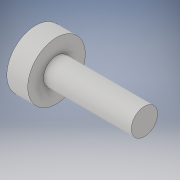
# Autodesk Inventor part: TableLEG
Saved by Autodesk Inventor 2018 (Build 220112000, 112)
## iProperties
Created: 2019-03-13
Part Number: TableLEG
Material: Generic
Document SubType Name: Modeling
Designer: 10043883
Density: 1 g/cm^3
Appearance: Default
Author: 10043883
Autodesk Inventor part; units mm, degrees
ref_plane "YZ Plane" through (0, 0, 0) normal (1, 0, 0) x (0, 1, 0)
ref_plane "XZ Plane" through (0, 0, 0) normal (0, 1, 0) x (-1, 0, 0)
ref_plane "XY Plane" through (0, 0, 0) normal (0, 0, 1) x (1, 0, 0)
sketch "Sketch1" plane through (0, 0, 0) normal (0, 0, 1) x (1, 0, 0)
  line L0 (-24.8503, 10.7907) -> (25.0184, 10.7907)
  line L1 (25.0184, 10.7907) -> (25.0184, 4.7721)
  line L2 (25.0184, 4.7721) -> (-15.2501, 4.7721)
  line L3 (-24.8503, -2.3863) -> (-24.8503, 10.7907)
  line L4 (-15.2501, 4.7721) -> (-15.2501, -2.3863)
  line L5 (-15.2501, -2.3863) -> (-24.8503, -2.3863)
  line L6 (-24.8503, -2.3863) -> (-24.8503, -2.3863)
  constraints: 14 end point, 2 parallel, 1 horizontal, 1 midpoint, 1 perpendicular, 1 point on line
revolve "Revolution1" add sketch "Sketch1" angle 360 about axis through (-24.8503, 10.7907, 0) along (1, 0, 0)
body "Solid1"
